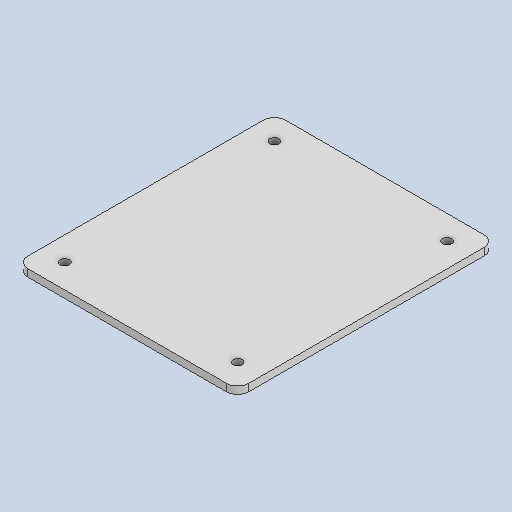
# Autodesk Inventor part: Kraicka_senzory_vrchnak
Saved by Autodesk Inventor 2025 (Build 290162000, 162)
## iProperties
Created: 2025-07-28
Part Number: Kraicka_senzory_vrchnak
Material: Generic
Document SubType Name: Modeling
Designer: Pravoslav
Density: 1 g/cm^3
Appearance: Default
Author: Pravoslav
Autodesk Inventor part; units mm, degrees
ref_plane "YZ Plane" through (0, 0, 0) normal (1, 0, 0) x (0, 1, 0)
ref_plane "XZ Plane" through (0, 0, 0) normal (0, 1, 0) x (-1, 0, 0)
ref_plane "XY Plane" through (0, 0, 0) normal (0, 0, 1) x (1, 0, 0)
sketch "Sketch1" plane through (0, 0, 0) normal (0, 1, 0) x (-1, 0, 0)
  line L0 (30, 35) -> (-30, 35)
  line L1 (-30, 35) -> (-30, -35)
  line L2 (-30, -35) -> (30, -35)
  line L3 (30, -35) -> (30, 35)
  line L4 (30, 35) -> (-30, -35) construction
  line L5 (-30, 35) -> (30, -35) construction
  point P0 (0, 0)
  dimension "d0" = 60
  dimension "d1" = 70
  constraints: 12 end point, 2 midpoint, 2 parallel, 1 horizontal, 1 perpendicular
  measures "d0" distance of L2.end L1.end
  measures "d1" distance of L1.end L0.end
extrude "Extrusion1" add sketch "Sketch1" along normal blind 2
sketch "Sketch2" plane through (0, 2, 0) normal (0, 1, 0) x (1, 0, 0)
  circle A0 centre (-23.5, -28.5) radius 1.25
  line L0 (-30, 35) -> (-30, -35) projected
  line L1 (-30, -35) -> (30, -35) projected
  point P0 (0, 0)
  dimension "d4" = 2.5
  dimension "d5" = 6.5
  dimension "d6" = 6.5
  constraints: 1 centre point
  measures "d4" diameter of A0
  measures "d5" distance from line of L0 A0.centre
  measures "d6" distance from line of L1 A0.centre
extrude "Extrusion2" cut sketch "Sketch2" against normal blind 2
mirror "Mirror1" about plane through (0, 0, 0) normal (0, 0, 1) of "Extrusion2"
mirror "Mirror2" about plane through (0, 0, 0) normal (1, 0, 0) of "Extrusion2", "Mirror1"
fillet "Fillet1" radius 3 4 edges at (-30, 1, 35) (-30, 1, -35) (30, 1, -35) (30, 1, 35)
body "Solid1"
